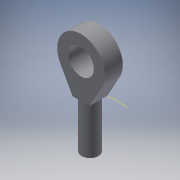
# Autodesk Inventor part: K
Saved by Autodesk Inventor 2019 (Build 230136000, 136)
## iProperties
Created: 2019-10-31
Part Number: K
Material: Generic
Document SubType Name: Modeling
Designer: Mark
Density: 1 g/cm^3
Appearance: Default
Author: Mark
Autodesk Inventor part; units mm, degrees
ref_plane "YZ Plane" through (0, 0, 0) normal (1, 0, 0) x (0, 1, 0)
ref_plane "XZ Plane" through (0, 0, 0) normal (0, 1, 0) x (-1, 0, 0)
ref_plane "XY Plane" through (0, 0, 0) normal (0, 0, 1) x (1, 0, 0)
sketch "Sketch1" plane through (0, 0, 0) normal (0, 1, 0) x (-1, 0, 0)
  circle A0 centre (0, 0.2739) radius 5
  point P0 (0, 0)
  dimension "d0" = 10
  constraints: 1 centre point
  measures "d0" diameter of A0
extrude "Extrusion1" add sketch "Sketch1" along normal blind 28
sketch "Sketch3" plane through (0, 28, 0.2739) normal (0, 1, 0) x (1, 0, 0)
  line L0 (14, -5.25) -> (-14, -5.25)
  line L1 (-14, -5.25) -> (-14, 5.25)
  line L2 (-14, 5.25) -> (14, 5.25)
  line L3 (14, 5.25) -> (14, -5.25)
  line L4 (14, -5.25) -> (-14, 5.25) construction
  line L5 (-14, -5.25) -> (14, 5.25) construction
  circle A0 centre (0, 0) radius 5 projected
  point P0 (0, 0.2739)
  point P1 (0, 0)
  dimension "d5" = 28
  dimension "d6" = 10.5
  dimension "d16" = 5.25
  constraints: 12 end point, 2 midpoint, 2 parallel, 1 horizontal, 1 perpendicular
  measures "d5" distance of L1.end L2.end
  measures "d6" distance of L0.end L1.end
  measures "d16" distance from line of A0.centre L2
extrude "Extrusion2" add sketch "Sketch3" along normal blind 34 contours L0 L1 L2 L3 | A0
sketch "Sketch4" plane through (-14, 28, 5.5239) normal (0, 0, 1) x (1, 0, 0)
  circle A0 centre (14, 20) radius 7.5
  line L0 (9, -28) -> (19, -28) projected
  line L1 (28, 0) -> (28, 34) projected
  circle A1 centre (14, 20) radius 14
  line L2 (19, 0) -> (9, 0) projected
  line L3 (9, 0) -> (1.7243, 13.2689)
  line L4 (19, -28) -> (19, 0) projected
  line L5 (19, 0) -> (26.2757, 13.2689)
  line L6 (19, 0) -> (28, 0)
  line L7 (28, 0) -> (28, 20)
  line L8 (28, 0) -> (0, 0) projected
  line L9 (0, 0) -> (9, 0)
  line L10 (0, 0) -> (0, 20)
  line L11 (0, 0) -> (0, 34) projected
  line L12 (0, 20) -> (0, 34)
  line L13 (0, 34) -> (14, 34)
  line L14 (0, 34) -> (28, 34) projected
  line L15 (14, 34) -> (28, 34)
  line L16 (28, 34) -> (28, 20)
  point P0 (14, -28)
  dimension "d9" = 15
  dimension "d10" = 48
  dimension "d11" = 14
  dimension "d12" = 28
  dimension "d13" = 13.2689
  constraints: 20 end point, 4 point on circle, 3 collinear, 3 point on line, 2 centre point, 2 tangent, 1 coincident, 1 horizontal, 1 midpoint, 1 perpendicular
  measures "d9" diameter of A0
  measures "d10" distance from line of L0 A0.centre
  measures "d11" distance from line of L1 A0.centre
  measures "d12" diameter of A1
  measures "d13" vertical distance of L5.start L5.end
extrude "Extrusion3" cut sketch "Sketch4" against normal blind 34 contours A0 | L6 L5 A1 L1 | A1 L14 L1 | A1 L11 L13 | L8 L10 A1 L3
body "Solid1"
